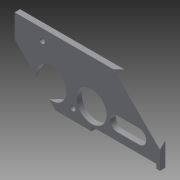
# Autodesk Inventor part: Yagi_Injector_Wall
Saved by Autodesk Inventor 2014 (Build 180170000, 170)
## iProperties
Created: 2015-01-07
Part Number: Yagi_Injector_Wall
Material: Generic
Document SubType Name: Modeling
Designer: Owner
Density: 1 g/cm^3
Appearance: Default
Author: Owner
Autodesk Inventor part; units mm, degrees
ref_plane "YZ Plane" through (0, 0, 0) normal (1, 0, 0) x (0, 1, 0)
ref_plane "XZ Plane" through (0, 0, 0) normal (0, 1, 0) x (-1, 0, 0)
ref_plane "XY Plane" through (0, 0, 0) normal (0, 0, 1) x (1, 0, 0)
sketch "Sketch1" plane through (0, 0, 0) normal (0, 0, 1) x (1, 0, 0)
  line L0 (-88.3152, 7.2276) -> (-2.5902, 7.2276)
  line L1 (-2.5902, 7.2276) -> (-2.5902, -30.8724)
  line L2 (-2.5902, -30.8724) -> (-88.3152, -30.8724)
  line L3 (-88.3152, -30.8724) -> (-88.3152, 7.2276)
  circle A0 centre (-72.1823, 0.7931) radius 1.5875
  circle A1 centre (-54.035, -24.4653) radius 1.5875
  circle A2 centre (-11.1215, 0.7931) radius 1.5875
  circle A3 centre (-66.6709, -18.1724) radius 8.89
  circle A4 centre (-42.9219, -18.1724) radius 8.89
  line L4 (-27.6819, -19.4424) -> (-14.9819, -19.4424) construction
  line L5 (-27.6819, -23.6758) -> (-14.9819, -23.6758)
  line L6 (-14.9819, -15.2091) -> (-27.6819, -15.2091)
  arc A5 (-27.6819, -15.2091) -> (-27.6819, -23.6758) centre (-27.6819, -19.4424) ccw
  arc A6 (-14.9819, -23.6758) -> (-14.9819, -15.2091) centre (-14.9819, -19.4424) ccw
  line L7 (-40.4323, 7.2276) -> (-15.0323, 7.2276)
  line L8 (-42.9219, -30.8724) -> (-4.8219, -30.8724)
  line L9 (-4.8219, -30.8724) -> (-4.8219, -28.3324)
  line L10 (-4.8219, -28.3324) -> (-42.9219, -28.3324)
  line L11 (-42.9219, -28.3324) -> (-42.9219, -30.8724)
  point P0 (0, 0)
  point P1 (-21.3319, -19.4424)
  dimension "d2" = 85.725
  dimension "d3" = 38.1
  dimension "d4" = 3.175
  dimension "d5" = 3.175
  dimension "d6" = 3.175
  dimension "d9" = 17.78
  dimension "d10" = 17.78
  dimension "d11" = 12.7
  dimension "d12" = 12.7
  dimension "d13" = 23.749
  dimension "d18" = 6.4345
  dimension "d19" = 6.4345
  dimension "d20" = 61.0608
  dimension "d21" = 6.4071
  dimension "d22" = 11.1131
  dimension "d23" = 5.5114
  dimension "d24" = 11.43
  dimension "d25" = 12.7
  dimension "d26" = 15.24
  dimension "d30" = 4.2333
  dimension "d31" = 2.54
  dimension "d32" = 38.1
  dimension "d33" = 0
  constraints: 26 end point, 7 centre point, 6 parallel, 4 point on circle, 4 tangent, 3 horizontal, 2 perpendicular, 2 point on line, 1 midpoint
  measures "d2" distance of L0.start L0.end
  measures "d3" distance of L0.end L1.end
  measures "d4" diameter of A0
  measures "d5" diameter of A2
  measures "d6" diameter of A1
  measures "d9" diameter of A4
  measures "d10" diameter of A3
  measures "d11" distance from line of L2 A3.centre
  measures "d12" distance from line of L2 A4.centre
  measures "d13" distance of A4.centre A3.centre
  measures "d18" distance from line of L0 A0.centre
  measures "d19" distance from line of L0 A2.centre
  measures "d20" distance of A0.centre A2.centre
  measures "d21" distance from line of L2 A1.centre
  measures "d22" horizontal distance of A4.centre A1.centre
  measures "d23" horizontal distance of A0.centre A3.centre
  measures "d24" distance between parallel lines of L2 L4
  measures "d25" distance of L4.start L4.end
  measures "d26" horizontal distance of A4.centre L4.start
  measures "d30" radius of A5
  measures "d31" distance of L10.end L8.start
  measures "d32" distance of L9.end L10.end
  measures "d33" distance from line of A4.centre L11
extrude "Extrusion1" add sketch "Sketch1" along normal blind 3.175 contours L0 L1 L2 L9 L10 L11 L3
body "Solid1"
